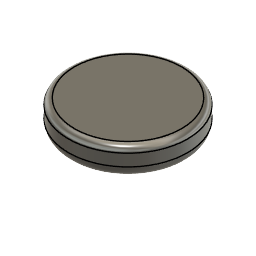
PrazdnyPIN (Autodesk Fusion 360 design; units mm, degrees)
Autodesk Fusion 360 part; units mm, degrees
sketch "Sketch6" plane through (0, 0, 0) normal (0, 1, 0) x (1, 0, 0)
  line L0 (0, 0) -> (5, 0)
  line L1 (5, 0) -> (5, 5)
  line L2 (5, 5) -> (0, 5)
  line L3 (0, 5) -> (0, 0)
  dimension "d136" = 5
  dimension "d137" = 5
  constraint horizontal L0
  constraint vertical L1
  constraint horizontal L2
  constraint vertical L3
  constraint coincident L0.start L3.end
  measures "d136" distance of L0.start L0.end
  measures "d137" distance of L0.start L2.end
extrude "Extrude25" add sketch "Sketch6" along normal blind 3.8
chamfer "Chamfer1" distance 1 angle 45 4 edges at (5, 0, -2.5) (2.5, 0, -5) (0, 0, -2.5) (2.5, 0, 0)
sketch "Sketch7" plane through (0, 3.8, 0) normal (0, 1, 0) x (-1, 0, 0)
  line L0 (0, -5) -> (0, 0)
  line L1 (0, 0) -> (-5, 0)
  line L2 (-5, 0) -> (-5, -5)
  line L3 (-5, -5) -> (0, -5)
  circle A0 centre (-2.5, -2.5) radius 10
  dimension "d141" = 20
  measures "d141" diameter of A0
extrude "Extrude26" add sketch "Sketch7" along normal blind 5 contours L0 L1 L2 L3 | A0
fillet "Fillet20" radius 2 1 edges at (11.8233, 3.8, -6.1162)
fillet "Fillet20" radius 1 1 edges at (11.8233, 8.8, -6.1162)
sketch "Sketch2" plane through (0, 6, 0) normal (0, 1, 0) x (-1, 0, 0)
  line L0 (0, -10) -> (0, 0)
  line L1 (0, 0) -> (-5, 0)
  line L2 (-5, 0) -> (-5, -10)
  line L3 (-5, -10) -> (0, -10)
  line L4 (-5, -7.5) -> (0, -7.5)
  line L5 (0, -7.5) -> (0, -2.5)
  line L6 (0, -2.5) -> (-5, -2.5)
  line L7 (-5, -2.5) -> (-5, -7.5)
  dimension "d98" = 5
  dimension "d99" = 5
  dimension "d100" = 2.5
  constraint horizontal L4
  constraint vertical L5
  constraint horizontal L6
  constraint vertical L7
  constraint collinear L2 L7
  measures "d98" distance of L4.start L4.end
  measures "d99" distance of L4.start L6.end
  measures "d100" distance of L3 L4
sketch "Sketch3" plane through (0, 12, 0) normal (0, 1, 0) x (-1, 0, 0)
  circle A0 centre (-2.5, -5) radius 10
  line L0 (-5, -2.5) -> (-5, -7.5)
  line L1 (-5, -7.5) -> (0, -7.5)
  line L2 (0, -7.5) -> (0, -2.5)
  line L3 (0, -2.5) -> (-5, -2.5)
  dimension "d10" = 20
  measures "d10" diameter of A0
extrude "Extrude3" [rolled back] along distance 5 taper angle 0
fillet "Fillet1" [rolled back] radius 2 radius 1
sketch "Sketch4" plane through (0, 17, 0) normal (0, 1, 0) x (-1, 0, 0)
  circle A0 centre (-2.5, -5) radius 9
  point P0 (-1.485, 3.5397)
combine "Combine2" [no effect]
move_body "Move2" [rolled back]
extrude "Extrude5" [suppressed]
extrude "Extrude6" [suppressed]
extrude "Extrude7" [suppressed]
fillet "Fillet2" [suppressed]
extrude "Extrude8" [suppressed]
fillet "Fillet3" [suppressed]
fillet "Fillet4" [suppressed]
extrude "Extrude9" [suppressed]
fillet "Fillet5" [suppressed]
extrude "Extrude10" [suppressed]
extrude "Extrude11" [suppressed]
extrude "Extrude12" [suppressed]
extrude "Extrude13" [suppressed]
extrude "Extrude14" [suppressed]
extrude "Extrude15" [suppressed]
fillet "Fillet6" [suppressed]
fillet "Fillet7" [suppressed]
fillet "Fillet8" [suppressed]
fillet "Fillet9" [suppressed]
fillet "Fillet10" [suppressed]
fillet "Fillet11" [suppressed]
extrude "Extrude4" [suppressed]
extrude "Extrude16" [suppressed]
extrude "Extrude17" [suppressed]
extrude "Extrude18" [suppressed]
extrude "Extrude19" [suppressed]
extrude "Extrude20" [suppressed]
fillet "Fillet12" [suppressed]
fillet "Fillet13" [suppressed]
fillet "Fillet14" [suppressed]
extrude "Extrude21" [suppressed]
extrude "Extrude22" [suppressed]
extrude "Extrude23" [suppressed]
fillet "Fillet15" [suppressed]
extrude "Extrude24" [suppressed]
fillet "Fillet16" [suppressed]
fillet "Fillet17" [suppressed]
fillet "Fillet18" [suppressed]
fillet "Fillet19" [suppressed]
combine "Combine1" [suppressed]
move_body "Move1" [suppressed]
